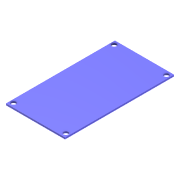
# Autodesk Inventor part: LM2596 Buck Converter
Saved by Autodesk Inventor 2022 (Build 260153000, 153)
## iProperties
Created: 2024-06-26
Part Number: LM2596 Buck Converter
Material: Generic
Document SubType Name: Modeling
Designer: david
Density: 1 g/cm^3
Appearance: Smooth - Dark Forest Green
Author: david
Autodesk Inventor part; units mm, degrees
ref_plane "YZ Plane" through (0, 0, 0) normal (1, 0, 0) x (0, 1, 0)
ref_plane "XZ Plane" through (0, 0, 0) normal (0, 1, 0) x (-1, 0, 0)
ref_plane "XY Plane" through (0, 0, 0) normal (0, 0, 1) x (1, 0, 0)
sketch "Sketch1" plane through (0, 0, 0) normal (0, 1, 0) x (-1, 0, 0)
  line L0 (18, -33.25) -> (-18, -33.25)
  line L1 (-18, -33.25) -> (-18, 33.25)
  line L2 (-18, 33.25) -> (18, 33.25)
  line L3 (18, 33.25) -> (18, -33.25)
  line L4 (18, -33.25) -> (-18, 33.25) construction
  line L5 (-18, -33.25) -> (18, 33.25) construction
  point P0 (0, 0)
  dimension "d0" = 36
  dimension "d1" = 66.5
  constraints: 12 end point, 2 midpoint, 2 parallel, 1 horizontal, 1 perpendicular
  measures "d0" distance of L1.end L2.end
  measures "d1" distance of L0.end L1.end
extrude "Extrusion1" add sketch "Sketch1" along normal blind 1
sketch "Sketch2" plane through (0, 1, 0) normal (0, 1, 0) x (1, 0, 0)
  line L0 (-18, -33.25) -> (-18, 33.25) projected
  line L1 (-18, 33.25) -> (18, 33.25) projected
  line L2 (18, 33.25) -> (18, -33.25) projected
  line L3 (18, -33.25) -> (-18, -33.25) projected
  line L4 (16, -30.75) -> (-16, -30.75) construction
  line L5 (-16, -30.75) -> (-16, 30.75) construction
  line L6 (-16, 30.75) -> (16, 30.75) construction
  line L7 (16, 30.75) -> (16, -30.75) construction
  line L8 (16, -30.75) -> (-16, 30.75) construction
  line L9 (-16, -30.75) -> (16, 30.75) construction
  circle A0 centre (-16, -30.75) radius 1.5 construction
  circle A1 centre (-16, 30.75) radius 1.5 construction
  circle A2 centre (16, -30.75) radius 1.5 construction
  circle A3 centre (16, 30.75) radius 1.5 construction
  point P0 (0, 0)
  point P1 (0, 0)
  dimension "d11" = 3
  dimension "d12" = 3
  dimension "d13" = 3
  dimension "d14" = 3
  dimension "d17" = 0.5
  dimension "d18" = 1
  constraints: 12 end point, 8 coincident, 4 centre point, 3 midpoint, 2 parallel, 1 horizontal, 1 perpendicular
  measures "d11" diameter of A1
  measures "d12" diameter of A0
  measures "d13" diameter of A2
  measures "d14" diameter of A3
  measures "d17" distance edge to line of A1 L0
  measures "d18" distance edge to line of A1 L1
hole "Hole1" at (-16, 1, 30.75) at (16, 1, 30.75) at (16, 1, -30.75) at (-16, 1, -30.75) direction (0, -1, 0) diameter 3 depth 6
equation "\"d12\" = d11"
equation "\"d13\" = d11"
equation "\"d14\" = d11"
body "Solid1"
